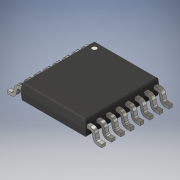
# Autodesk Inventor part: Semiconductor_TSSOP-16
Saved by Autodesk Inventor 2018 (Build 220112000, 112)
## iProperties
Created: 2016-07-22
Part Number: Semiconductor_TSSOP-16
Material: ABS Plastic
Document SubType Name: Modeling
Designer: Bradley
Density: 1.06 g/cm^3
Appearance: Smooth - Black
Mass: 0.00993513 g
Surface Area: 0.40182 cm^2
Volume: 0.00937276 cm^3
Author: Bradley
Autodesk Inventor part; units mm, degrees
ref_plane "YZ Plane" through (0, 0, 0) normal (1, 0, 0) x (0, 1, 0)
ref_plane "XZ Plane" through (0, 0, 0) normal (0, 1, 0) x (-1, 0, 0)
ref_plane "XY Plane" through (0, 0, 0) normal (0, 0, 1) x (1, 0, 0)
sketch "Sketch1" plane through (0, 0, 0) normal (0, 1, 0) x (-1, 0, 0)
  line L0 (-2.2, 2.5) -> (2.2, 2.5)
  line L1 (2.2, 2.5) -> (2.2, -2.5)
  line L2 (2.2, -2.5) -> (-2.2, -2.5)
  line L3 (-2.2, -2.5) -> (-2.2, 2.5)
  line L4 (-2.2, 2.5) -> (2.2, -2.5) construction
  line L5 (2.2, 2.5) -> (-2.2, -2.5) construction
  point P0 (0, 0)
  dimension "d0" = 4.4
  dimension "d1" = 5
  constraints: 12 end point, 2 midpoint, 2 parallel, 1 horizontal, 1 perpendicular
  measures "d0" distance of L1.end L2.end
  measures "d1" distance of L0.end L1.end
extrude "Extrusion1" add sketch "Sketch1" along normal blind 0.55 draft -5
sketch "Sketch2" plane through (0, 0, 0) normal (0, -1, 0) x (1, 0, 0)
  line L0 (2.2, 2.5) -> (-2.2, 2.5) projected
  line L1 (2.2, 2.5) -> (-2.2, 2.5) projected
  line L2 (-2.2, 2.5) -> (-2.2, -2.5) projected
  line L3 (-2.2, -2.5) -> (2.2, -2.5) projected
  line L4 (2.2, -2.5) -> (2.2, 2.5) projected
  point P0 (0, 0)
extrude "Extrusion2" add sketch "Sketch2" along normal blind 0.55 draft -5
fillet "Fillet1" radius 0.1 8 edges at (-2.1519, 0.55, 0) (0, 0.55, 2.4519) (0, 0.55, -2.4519) (2.1519, 0.55, 0) (2.1519, -0.55, 0) (0, -0.55, 2.4519) (-2.1519, -0.55, 0) (0, -0.55, -2.4519)
sketch "Sketch3" plane through (0, 0, 0) normal (0, 1, 0) x (-1, 0, 0)
  line L0 (2.2, 2.5) -> (2.2, -2.5) projected
  line L1 (-2.2, 2.5) -> (2.2, 2.5) projected
  line L2 (2.2, 2.4) -> (2.4, 2.4)
  line L3 (2.4, 2.4) -> (2.4, 2.15)
  line L4 (2.4, 2.15) -> (2.2, 2.15)
  line L5 (2.2, 2.15) -> (2.2, 2.4)
  line L6 (-2.2, -2.5) -> (-2.2, 2.5) projected
  line L7 (-2.2, 2.4) -> (-2.4, 2.4)
  line L8 (-2.4, 2.4) -> (-2.4, 2.15)
  line L9 (-2.4, 2.15) -> (-2.2, 2.15)
  line L10 (-2.2, 2.15) -> (-2.2, 2.4)
  line L11 (-2.2, 2.15) -> (2.2, 2.15)
  line L12 (2.2, 2.15) -> (2.2, 2.4)
  line L13 (2.2, 2.4) -> (-2.2, 2.4)
  line L14 (-2.2, 2.4) -> (-2.2, 2.15)
  point P0 (0, 0)
  point P1 (2.2, 2.275)
  dimension "d7" = 0.25
  dimension "d8" = 2.275
  dimension "d9" = 0.2
  constraints: 24 end point, 6 parallel, 4 point on line, 3 horizontal, 3 perpendicular, 1 collinear, 1 midpoint
  measures "d7" distance of L2.end L3.end
  measures "d8" vertical distance of point (2.2, 2.275) point (0, 0)
  measures "d9" distance of L3.end L4.end
extrude "Extrusion3" add sketch "Sketch3" along normal blind 0.2 contours L2 L3 L4 L0 | L0 L11 L6 L13 | L6 L9 L8 L7
sketch "Sketch4" plane through (-2.4, 0, 2.4) normal (0, 0, 1) x (1, 0, 0)
  line L0 (0.2175, 0.2) -> (0.2, 0) projected
  line L1 (0, 0.2) -> (0.2175, 0.2) projected
  line L2 (0, 0) -> (0, 0.2) projected
  line L3 (0, 0) -> (0.2, 0) projected
  line L4 (4.6, 0) -> (4.5825, 0.2) projected
  line L5 (4.6, 0) -> (4.8, 0) projected
  line L6 (4.8, 0) -> (4.8, 0.2) projected
  line L7 (4.5825, 0.2) -> (4.8, 0.2) projected
  line L8 (0, 0) -> (0.2, 0) projected
  arc A0 (0, 0) -> (-0.1468, -0.1191) centre (0, -0.15) ccw
  arc A1 (-0.5425, -0.65) -> (-0.2, -0.3721) centre (-0.5425, -0.3) ccw
  line L9 (0, 0.2) -> (0.2175, 0.2) projected
  arc A2 (0, 0.2) -> (-0.3425, -0.0779) centre (0, -0.15) ccw
  arc A3 (-0.5425, -0.45) -> (-0.3957, -0.3309) centre (-0.5425, -0.3) ccw
  line L10 (-0.5425, -0.65) -> (-0.8, -0.65)
  line L11 (-0.8, -0.65) -> (-0.8, -0.45)
  line L12 (-0.8, -0.45) -> (-0.5425, -0.45)
  line L13 (-0.3425, -0.0779) -> (-0.3957, -0.3309)
  line L14 (-0.1468, -0.1191) -> (-0.2, -0.3721)
  line L15 (4.4602, -0.55) -> (0.3398, -0.55) projected
  line L16 (0, 0.2) -> (0, 0)
  line L17 (0.3398, 0.55) -> (4.4602, 0.55) projected
  line L18 (2.4, 0.5) -> (2.4, -0.5)
  line L19 (4.8, 0) -> (4.8, 0.2)
  arc A4 (4.9468, -0.1191) -> (4.8, 0) centre (4.8, -0.15) ccw
  arc A5 (5, -0.3721) -> (5.3425, -0.65) centre (5.3425, -0.3) ccw
  arc A6 (5.1425, -0.0779) -> (4.8, 0.2) centre (4.8, -0.15) ccw
  arc A7 (5.1957, -0.3309) -> (5.3425, -0.45) centre (5.3425, -0.3) ccw
  line L20 (5.3425, -0.65) -> (5.6, -0.65)
  line L21 (5.6, -0.65) -> (5.6, -0.45)
  line L22 (5.6, -0.45) -> (5.3425, -0.45)
  line L23 (5.1425, -0.0779) -> (5.1957, -0.3309)
  line L24 (4.9468, -0.1191) -> (5, -0.3721)
  point P0 (2.4, 0)
  dimension "d12" = 0.15
  dimension "d13" = 0.15
  dimension "d16" = 0.6
  dimension "d17" = 0.1
  dimension "d25" = 6.4
  constraints: 26 end point, 16 point on circle, 12 symmetric about line, 8 centre point, 6 tangent, 4 coincident, 2 equal length, 2 perpendicular, 1 horizontal, 1 parallel, 4 other
  measures "d12" radius of A0
  measures "d13" radius of A3
  measures "d16" distance from line of L11 L14.end
  measures "d17" distance between parallel lines of L10 L15
  measures "d25" distance between parallel lines of L21 L11
extrude "Extrusion4" add sketch "Sketch4" against normal up to surface (0.25 mm away) contours L2 A0 L14 A1 L10 L11 L12 A3 L13 A2 | L6 A6 L23 A7 L22 L21 L20 A5 L24 A4
pattern_linear "Rectangular Pattern1" count 8 spacing 0.65 along (0, 0, -1) of "Extrusion4", "Extrusion3"
sketch "Sketch5" plane through (0, 0.55, 0) normal (0, 1, 0) x (1, 0, 0)
  line L0 (2.0602, -2.3602) -> (-2.0602, -2.3602) projected
  line L1 (2.0602, 2.3602) -> (2.0602, -2.3602) projected
  line L2 (-2.0602, 2.3602) -> (2.0602, 2.3602) projected
  line L3 (-2.0602, -2.3602) -> (-2.0602, 2.3602) projected
  circle A0 centre (-1.7, 2) radius 0.15
  circle A1 centre (-1.7, 2) radius 0.3602 construction
  line L4 (-2.0602, -2.3602) -> (-2.0602, 2.3602) projected
  line L5 (-2.0602, -2.3602) -> (2.0602, -2.3602) construction
  line L6 (-2.0602, 2.3602) -> (2.0602, 2.3602) construction
  line L7 (-2.2, 2.5) -> (2.2, 2.5) projected
  point P0 (0, 0)
  dimension "d26" = 0.5
  dimension "d27" = 0.3
  constraints: 2 centre point, 2 tangent, 1 coincident
  measures "d26" distance from line of A0.centre L7
  measures "d27" diameter of A0
extrude "Extrusion5" add sketch "Sketch5" along normal blind 0.01 and the other way blind 0.255 contours A0
equation "\"d13\" = d12"
body "Solid1"
